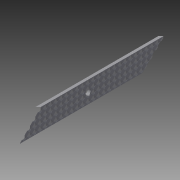
# Autodesk Inventor part: rubber grip
Saved by Autodesk Inventor 2015 SP1 (Build 190203100, 203)
## iProperties
Created: 2015-02-05
Part Number: rubber grip
Material: Generic
Document SubType Name: Modeling
Designer: Admin
Density: 1 g/cm^3
Appearance: Default
Author: Admin
Autodesk Inventor part; units mm, degrees
ref_plane "YZ Plane" through (0, 0, 0) normal (1, 0, 0) x (0, 1, 0)
ref_plane "XZ Plane" through (0, 0, 0) normal (0, 1, 0) x (-1, 0, 0)
ref_plane "XY Plane" through (0, 0, 0) normal (0, 0, 1) x (1, 0, 0)
sketch "Sketch1" plane through (0, 0, 0) normal (1, 0, 0) x (0, 1, 0)
  line L0 (0, 0) -> (25.4, 0)
  line L1 (25.4, 0) -> (25.4, -184.15)
  line L2 (25.4, -184.15) -> (0, -184.15)
  line L3 (0, -184.15) -> (0, 0)
  dimension "d0" = 25.4
  dimension "d1" = 184.15
  constraints: 8 end point, 2 parallel, 1 horizontal, 1 perpendicular
  measures "d0" distance of L1.end L2.end
  measures "d1" distance of L0.end L1.end
extrude "Extrusion1" add sketch "Sketch1" along normal blind 3.175
sketch "Sketch2" plane through (3.175, 0, 0) normal (1, 0, 0) x (0, 0, -1)
  line L0 (0, 25.4) -> (3.175, 25.4) construction
  line L1 (3.175, 25.4) -> (3.175, 0) construction
  line L2 (3.175, 0) -> (0, 0) construction
  line L3 (0, 0) -> (0, 25.4) construction
  line L4 (3.175, 25.4) -> (6.35, 25.4) construction
  line L5 (6.35, 25.4) -> (6.35, 0) construction
  line L6 (6.35, 0) -> (3.175, 0) construction
  line L7 (3.175, 0) -> (3.175, 25.4) construction
  line L8 (3.175, 25.4) -> (0, 22.225)
  line L9 (3.175, 25.4) -> (7.6651, 25.4) construction
  line L10 (0, 22.225) -> (3.175, 19.05)
  line L11 (0, 22.225) -> (4.4901, 22.225) construction
  line L12 (3.175, 19.05) -> (0, 15.875)
  line L13 (0, 15.875) -> (3.175, 12.7)
  line L14 (3.175, 12.7) -> (0, 9.525)
  line L15 (3.175, 12.7) -> (7.6651, 12.7) construction
  line L16 (0, 9.525) -> (3.175, 6.35)
  line L17 (3.175, 6.35) -> (0, 3.175)
  line L18 (0, 3.175) -> (3.175, 0)
  line L19 (3.175, 25.4) -> (6.35, 22.225)
  line L20 (6.35, 22.225) -> (3.175, 19.05)
  line L21 (3.175, 19.05) -> (6.35, 15.875)
  line L22 (6.35, 15.875) -> (3.175, 12.7)
  line L23 (3.175, 12.7) -> (6.35, 9.525)
  line L24 (6.35, 9.525) -> (3.175, 6.35)
  line L25 (3.175, 6.35) -> (6.35, 3.175)
  line L26 (6.35, 3.175) -> (3.175, 0)
  dimension "d4" = 3.175
  dimension "d5" = 25.4
  dimension "d6" = 3.175
  dimension "d7" = 25.4
  dimension "d8" = 135
  dimension "d9" = 45
  dimension "d10" = 90
  dimension "d11" = 135
  dimension "d12" = 90
  dimension "d13" = 90
  constraints: 54 end point, 14 point on line, 5 horizontal, 4 parallel, 3 equal length, 2 perpendicular, 1 midpoint
  measures "d4" distance of L1.end L2.end
  measures "d5" distance of L0.end L1.end
  measures "d6" distance of L5.end L6.end
  measures "d7" distance of L4.end L5.end
  measures "d8" angle of L8 L9
  measures "d9" angle of L10 L11
  measures "d10" angle of L10 L12
  measures "d11" angle of L14 L15
  measures "d12" angle of L16 L14
  measures "d13" angle of L16 L17
extrude "Extrusion2" add sketch "Sketch2" along normal blind 1.5875 draft -60
pattern_linear "Rectangular Pattern1" count 29 spacing 6.35 along (0, 0, -1) of "Extrusion2"
sketch "Sketch3" plane through (0, 0, 0) normal (-1, 0, 0) x (0, 0, 1)
  line L0 (0, 0) -> (0, 25.4) projected
  line L1 (0, 25.4) -> (-184.15, 25.4) projected
  line L2 (-184.15, 25.4) -> (-184.15, 0) projected
  point P0 (-171.45, 12.7)
  point P1 (-92.075, 12.7)
  point P2 (-12.7, 12.7)
  dimension "d19" = 12.7
  dimension "d20" = 12.7
  dimension "d21" = 12.7
  dimension "d22" = 92.075
  dimension "d23" = 12.7
  dimension "d24" = 12.7
  measures "d19" distance from line of L1 point (-171.45, 12.7)
  measures "d20" distance from line of L2 point (-171.45, 12.7)
  measures "d21" distance from line of L1 point (-92.075, 12.7)
  measures "d22" distance from line of L2 point (-92.075, 12.7)
  measures "d23" distance from line of L0 point (-12.7, 12.7)
  measures "d24" distance from line of L1 point (-12.7, 12.7)
hole "Hole1" at (0, 12.7, -171.45) at (0, 12.7, -92.075) at (0, 12.7, -12.7) direction (1, 0, 0) diameter 6.35 end through all
body "Solid1"
